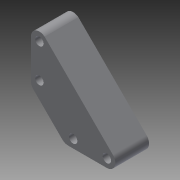
# Autodesk Inventor part: Corner
Saved by Autodesk Inventor 2014 (Build 180170000, 170)
## iProperties
Created: 2014-01-06
Part Number: Corner
Material: Generic
Document SubType Name: Modeling
Designer: Tristan Debrunner
Density: 1 g/cm^3
Appearance: Default
Author: Tristan Debrunner
Autodesk Inventor part; units mm, degrees
ref_plane "YZ Plane" through (0, 0, 0) normal (1, 0, 0) x (0, 1, 0)
ref_plane "XZ Plane" through (0, 0, 0) normal (0, 1, 0) x (-1, 0, 0)
ref_plane "XY Plane" through (0, 0, 0) normal (0, 0, 1) x (1, 0, 0)
sketch "Sketch1" plane through (0, 0, 0) normal (0, 0, 1) x (1, 0, 0)
  line L0 (21.6803, -6.35) -> (50.8, -6.35)
  arc A0 (50.8, -6.35) -> (55.2876, 4.4927) centre (50.8, 0) ccw
  line L1 (-4.4901, 17.1901) -> (17.1901, -4.4901)
  line L2 (-6.35, 21.6803) -> (-6.35, 50.8)
  arc A1 (4.9675, 54.7556) -> (-6.35, 50.8) centre (0, 50.8) ccw
  line L3 (3.9499, 55.772) -> (55.2876, 4.4927)
  arc A2 (-6.35, 21.6803) -> (-4.4901, 17.1901) centre (0, 21.6803) ccw
  arc A3 (17.1901, -4.4901) -> (21.6803, -6.35) centre (21.6803, 0) ccw
  circle A4 centre (0, 50.8) radius 3.175
  circle A5 centre (0, 25.4) radius 3.175
  circle A6 centre (25.4, 0) radius 3.175
  circle A7 centre (50.8, 0) radius 3.175
  point P0 (0, 0)
  dimension "d6" = 6.35
  dimension "d7" = 6.35
  dimension "d8" = 6.35
  dimension "d9" = 6.35
  dimension "d10" = 6.35
  constraints: 9 point on circle, 8 centre point, 8 end point, 6 coincident, 5 tangent, 1 equal radius, 1 perpendicular, 1 point on line
  measures "d6" radius of A2
  measures "d7" diameter of A4
  measures "d8" diameter of A5
  measures "d9" diameter of A6
  measures "d10" diameter of A7
extrude "Extrusion1" add sketch "Sketch1" along normal blind 25.4 contours A3 L1 A2 L2 A1 L3 A0 L0
body "Solid1"
